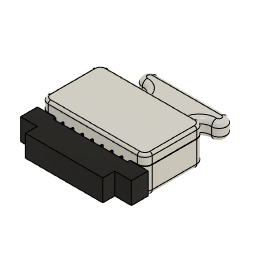
CBM8296_CP_Dongle v1 (Autodesk Fusion 360 design; units mm, degrees)
Autodesk Fusion 360 part; units mm, degrees
sketch "PCB" plane through (0, 0, 0) normal (0, 0, 1) x (1, 0, 0) in component "PCB"
  line L0 (30, 21) -> (0, 21)
  line L1 (0, 21) -> (0, 0)
  line L2 (0, 0) -> (30, 0)
  line L3 (30, 0) -> (30, 21)
  line L4 (2.87, 0) -> (2.87, -1)
  line L5 (19.05, 9.8425) -> (11.43, 9.8425)
  line L6 (7.33, -1) -> (7.33, 0)
  line L7 (25.9, 0.1) -> (25.9, -1)
  line L8 (15.98, 0.1) -> (15.98, -1)
  line L9 (-4.12, 0) -> (-5.82, 0)
  line L10 (11.43, 8.5725) -> (10.668, 8.5725)
  line L11 (14.75, 0) -> (14.75, -1)
  circle A0 centre (4, 12) radius 1.7463
  line L12 (15.25, 0) -> (14.75, 0)
  line L13 (14.02, 0.1) -> (14.02, -1)
  line L14 (23.17, 0) -> (22.67, 0)
  line L15 (8.06, 0.1) -> (8.06, -1)
  circle A1 centre (26, 12) radius 3.1789
  line L16 (3.37, 0) -> (2.87, 0)
  line L17 (19.21, -1) -> (19.21, 0)
  line L18 (10.06, 0.1) -> (10.06, -1)
  line L19 (6.1, 0.1) -> (6.1, -1)
  line L20 (0.08, -1) -> (0.08, 0)
  line L21 (-2.42, -6.8) -> (-2.42, -5.2)
  line L22 (15.25, -1) -> (15.25, 0)
  line L23 (4.1, 0.1) -> (4.1, -1)
  line L24 (19.21, 0) -> (18.71, 0)
  line L25 (26.63, 0) -> (26.63, -1)
  line L26 (18.71, 0) -> (18.71, -1)
  line L27 (29.92, -1) -> (0.08, -1)
  line L28 (-4.12, -7.9147) -> (-4.12, -8.052)
  line L29 (11.43, 9.8425) -> (11.43, 7.3025)
  line L30 (34.12, 0) -> (32.42, 0)
  line L31 (23.17, -1) -> (23.17, 0)
  line L32 (6.83, 0) -> (6.83, -1)
  line L33 (-4.12, -3.548) -> (-4.12, -3.6853)
  line L34 (23.9, 0.1) -> (23.9, -1)
  line L35 (37.37, 0) -> (35.82, 0)
  circle A2 centre (4, 12) radius 3.1789
  line L36 (12.02, 0.1) -> (12.02, -1)
  line L37 (7.33, 0) -> (6.83, 0)
  line L38 (27.13, -1) -> (27.13, 0)
  line L39 (11.29, 0) -> (10.79, 0)
  line L40 (10.79, 0) -> (10.79, -1)
  line L41 (-5.82, -6.8) -> (-7.37, -6.8)
  line L42 (11.43, 10.4775) -> (19.05, 10.4775)
  line L43 (-4.12, -4.3667) -> (-4.12, -7.2333)
  line L44 (11.29, -1) -> (11.29, 0)
  line L45 (19.94, 0.1) -> (19.94, -1)
  line L46 (27.13, 0) -> (26.63, 0)
  line L47 (3.37, -1) -> (3.37, 0)
  circle A3 centre (26, 12) radius 1.7463
  line L48 (17.98, 0.1) -> (17.98, -1)
  line L49 (37.37, 0) -> (37.37, -6.8)
  line L50 (21.94, 0.1) -> (21.94, -1)
  line L51 (22.67, 0) -> (22.67, -1)
  line L52 (35.82, -6.8) -> (32.42, -6.8)
  line L53 (0.08, 0) -> (-2.42, 0)
  line L54 (-5.82, 0) -> (-7.37, 0)
  line L55 (32.42, -4.2) -> (32.42, -2.6)
  line L56 (35.82, 0) -> (34.12, 0)
  line L57 (35.82, -4.2) -> (35.82, -2.6)
  line L58 (35.82, -6.8) -> (35.82, -5.2)
  line L59 (-4.12, 0) -> (-4.12, -2.8667)
  line L60 (30.62, -11.6) -> (-0.62, -11.6)
  line L61 (19.05, 8.5725) -> (19.812, 8.5725)
  line L62 (-0.62, -11.6) -> (-0.62, -6.8)
  line L63 (19.05, 11.7475) -> (19.812, 11.7475)
  line L64 (34.12, -3.6853) -> (34.12, -3.548)
  line L65 (34.12, -2.8667) -> (34.12, 0)
  line L66 (-2.42, -6.8) -> (-5.82, -6.8)
  line L67 (11.43, 13.0175) -> (11.43, 10.4775)
  line L68 (37.37, -6.8) -> (35.82, -6.8)
  line L69 (34.12, -11.6) -> (34.12, -8.7333)
  line L70 (11.43, 11.7475) -> (10.668, 11.7475)
  line L71 (34.12, -7.2333) -> (34.12, -4.3667)
  line L72 (-5.82, -1.6) -> (-5.82, 0)
  line L73 (-5.82, -4.2) -> (-5.82, -2.6)
  line L74 (34.12, -8.052) -> (34.12, -7.9147)
  line L75 (19.05, 10.4775) -> (19.05, 13.0175)
  line L76 (32.42, -6.8) -> (32.42, -5.2)
  line L77 (-2.42, -4.2) -> (-2.42, -2.6)
  line L78 (-7.37, 0) -> (-7.37, -6.8)
  line L79 (19.05, 7.3025) -> (19.05, 9.8425)
  line L80 (32.42, 0) -> (29.92, 0)
  line L81 (29.92, 0) -> (29.92, -1)
  line L82 (30.62, -6.8) -> (30.62, -11.6)
  line L83 (-4.12, -8.7333) -> (-4.12, -11.6)
  line L84 (35.82, -1.6) -> (35.82, 0)
  line L85 (-2.42, -1.6) -> (-2.42, 0)
  line L86 (32.42, -6.8) -> (30.62, -6.8)
  line L87 (11.43, 7.3025) -> (19.05, 7.3025)
  line L88 (-5.82, -6.8) -> (-5.82, -5.2)
  line L89 (32.42, -1.6) -> (32.42, 0)
  line L90 (-2.42, 0) -> (-4.12, 0)
  line L91 (19.05, 13.0175) -> (11.43, 13.0175)
  line L92 (-0.62, -6.8) -> (-2.42, -6.8)
  line L93 (25.9, 0.1) -> (25.9, 4)
  line L94 (25.4, 3) -> (25.4, 2)
  line L95 (4.6, 3) -> (4.6, 2)
  line L96 (6.1, 0.1) -> (6.1, 4)
  line L97 (13.52, 3) -> (13.52, 2)
  arc A4 (14.02, 4) -> (12.02, 4) centre (13.02, 4) ccw
  line L98 (17.48, 3) -> (17.48, 2)
  line L99 (10.06, 0.1) -> (10.06, 4)
  line L100 (23.9, 0.1) -> (23.9, 4)
  arc A5 (25.4, 3) -> (24.4, 3) centre (24.9, 3) ccw
  arc A6 (20.44, 2) -> (21.44, 2) centre (20.94, 2) ccw
  line L101 (21.44, 3) -> (21.44, 2)
  arc A7 (8.56, 2) -> (9.56, 2) centre (9.06, 2) ccw
  line L102 (4.1, 0.1) -> (4.1, 4)
  arc A8 (25.9, 4) -> (23.9, 4) centre (24.9, 4) ccw
  line L103 (24.4, 3) -> (24.4, 2)
  line L104 (14.02, 0.1) -> (14.02, 4)
  arc A9 (13.52, 3) -> (12.52, 3) centre (13.02, 3) ccw
  arc A10 (24.4, 2) -> (25.4, 2) centre (24.9, 2) ccw
  arc A11 (9.56, 3) -> (8.56, 3) centre (9.06, 3) ccw
  arc A12 (17.48, 3) -> (16.48, 3) centre (16.98, 3) ccw
  line L105 (16.48, 3) -> (16.48, 2)
  line L106 (9.56, 3) -> (9.56, 2)
  line L107 (17.98, 0.1) -> (17.98, 4)
  arc A13 (17.98, 4) -> (15.98, 4) centre (16.98, 4) ccw
  line L108 (12.52, 3) -> (12.52, 2)
  line L109 (19.94, 0.1) -> (19.94, 4)
  arc A14 (16.48, 2) -> (17.48, 2) centre (16.98, 2) ccw
  arc A15 (21.94, 4) -> (19.94, 4) centre (20.94, 4) ccw
  arc A16 (6.1, 4) -> (4.1, 4) centre (5.1, 4) ccw
  arc A17 (4.6, 2) -> (5.6, 2) centre (5.1, 2) ccw
  line L110 (20.44, 3) -> (20.44, 2)
  arc A18 (5.6, 3) -> (4.6, 3) centre (5.1, 3) ccw
  line L111 (8.56, 3) -> (8.56, 2)
  line L112 (5.6, 3) -> (5.6, 2)
  line L113 (12.02, 0.1) -> (12.02, 4)
  arc A19 (21.44, 3) -> (20.44, 3) centre (20.94, 3) ccw
  line L114 (8.06, 0.1) -> (8.06, 4)
  arc A20 (10.06, 4) -> (8.06, 4) centre (9.06, 4) ccw
  arc A21 (12.52, 2) -> (13.52, 2) centre (13.02, 2) ccw
  line L115 (15.98, 0.1) -> (15.98, 4)
  line L116 (21.94, 0.1) -> (21.94, 4)
extrude "Extrude1" add sketch "PCB" against normal blind 1.6 contours L0 L1 L2 L3 L7 L8 L12 L13 L14 L15 L16 L18 L19 L23 L24 L34 L36 L37 L39 L45 L46 L48 L50 L53 L80 L93 L96 A4 L99 L100 L102 A8 L104 L107 A13 L109 A15 A16 L113 L114 A20 L115 L116 | L2 L7 L34 L93 L100 A8 | L2 L19 L23 L96 L102 A16 | L2 L45 L50 L109 A15 L116 | L2 L15 L18 L99 L114 A20 | L2 L8 L48 L107 A13 L115 | L2 L13 L36 A4 L104 L113 | L5 L29 L79 L87 | A1 | A2 | L42 L67 L75 L91 | L94 A5 L103 A10 | L95 A17 A18 L112 | L97 A9 L108 A21 | L98 A12 L105 A14 | A6 L101 L110 A19 | A7 A11 L106 L111 makes body 1 in component "PCB"
extrude "Extrude9" add sketch "PCB" along normal blind 4.3 and the other way blind 4.4 contours L2 L9 L20 L27 L30 L35 L41 L49 L52 L53 L54 L56 L60 L62 L66 L68 L78 L80 L81 L82 L86 L90 L92 | L2 L25 L27 L38 L46 | L2 L4 L16 L27 L47 | L2 L14 L27 L31 L51 | L2 L6 L27 L32 L37 | L2 L17 L24 L26 L27 | L2 L27 L39 L40 L44 | L2 L11 L12 L22 L27 bodies 1 in component "PCB"
extrude "Extrude10" add sketch "PCB" along normal blind 0.5 contours L2 L7 L27 L34 | L2 L7 L34 L93 L100 A8 | L2 L19 L23 L96 L102 A16 | L2 L19 L23 L27 | L2 L27 L45 L50 | L2 L45 L50 L109 A15 L116 | L2 L15 L18 L99 L114 A20 | L2 L15 L18 L27 | L2 L8 L27 L48 | L2 L8 L48 L107 A13 L115 | L2 L13 L36 A4 L104 L113 | L2 L13 L27 L36 bodies 1 in component "PCB"
extrude "Extrude11" add sketch "PCB" against normal blind 0.5 from surface at -1.6 contours L2 L7 L27 L34 | L2 L7 L34 L93 L100 A8 | L2 L19 L23 L96 L102 A16 | L2 L19 L23 L27 | L2 L27 L45 L50 | L2 L45 L50 L109 A15 L116 | L2 L15 L18 L99 L114 A20 | L2 L15 L18 L27 | L2 L8 L27 L48 | L2 L8 L48 L107 A13 L115 | L2 L13 L36 A4 L104 L113 | L2 L13 L27 L36 bodies 1 in component "PCB"
ref_plane "WorkPlane1" through (0, 0, -4.4) normal (0, 0, 1) x (1, 0, 0) in component "bottom_shell"
sketch "bottom" plane through (0, 0, -4.4) normal (0, 0, 1) x (1, 0, 0) in component "bottom_shell"
  line L0 (15, 19.9973) -> (15, -5.0027) construction
  circle A0 centre (26, 12) radius 1.75
  circle A1 centre (4, 12) radius 1.75
  line L1 (36, 2.9752) -> (36, 20.9752)
  line L2 (-6, 2.9752) -> (-6, 20.9752)
  line L3 (33, 23.9752) -> (-3, 23.9752)
  line L4 (33, -0.0248) -> (-3, -0.0248)
  arc A2 (33, -0.0248) -> (36, 2.9752) centre (33, 2.9752) ccw
  arc A3 (36, 20.9752) -> (33, 23.9752) centre (33, 20.9752) ccw
  arc A4 (-3, 23.9752) -> (-6, 20.9752) centre (-3, 20.9752) ccw
  arc A5 (-6, 2.9752) -> (-3, -0.0248) centre (-3, 2.9752) ccw
  line L5 (33, 21.9752) -> (-3, 21.9752)
  arc A6 (-3, 21.9752) -> (-4, 20.9752) centre (-3, 20.9752) ccw
  line L6 (-4, 2.9752) -> (-4, 20.9752)
  arc A7 (-4, 2.9752) -> (-3, 1.9752) centre (-3, 2.9752) ccw
  line L7 (33, 1.9752) -> (-3, 1.9752)
  arc A8 (33, 1.9752) -> (34, 2.9752) centre (33, 2.9752) ccw
  line L8 (34, 2.9752) -> (34, 20.9752)
  arc A9 (34, 20.9752) -> (33, 21.9752) centre (33, 20.9752) ccw
  circle A10 centre (26, 12) radius 4.25
  circle A11 centre (4, 12) radius 4.25
  line L9 (30.6, 1.1752) -> (30.6, 1.9752)
  line L10 (-0.6, -0.0248) -> (-0.6, 1.9752)
  circle A12 centre (26, 12) radius 3
  circle A13 centre (4, 12) radius 3
  line L11 (33, 22.7752) -> (-3, 22.7752)
  arc A14 (-3, 22.7752) -> (-4.8, 20.9752) centre (-3, 20.9752) ccw
  line L12 (-4.8, 2.9752) -> (-4.8, 20.9752)
  arc A15 (-4.8, 2.9752) -> (-3, 1.1752) centre (-3, 2.9752) ccw
  arc A16 (33, 1.1752) -> (34.8, 2.9752) centre (33, 2.9752) ccw
  line L13 (34.8, 2.9752) -> (34.8, 20.9752)
  arc A17 (34.8, 20.9752) -> (33, 22.7752) centre (33, 20.9752) ccw
  line L14 (33, 1.1752) -> (30.6, 1.1752)
  line L15 (-0.6, 1.1752) -> (-3, 1.1752)
  line L16 (30.6, 1.1752) -> (30.6, -0.0248)
  line L17 (29, 28.9752) -> (29, 33.9752) construction
  line L18 (29, 33.9752) -> (1, 33.9752) construction
  line L19 (29, 33.9752) -> (29, 39.501) construction
  arc A18 (29, 33.9752) -> (29, 39.9752) centre (29, 36.9752) ccw
  arc A19 (29, 33.9752) -> (29, 23.9752) centre (29, 28.9752) ccw
  arc A20 (1, 23.9752) -> (1, 33.9752) centre (1, 28.9752) ccw
  line L20 (0, 21) -> (0, 0) construction
  line L21 (30, 0) -> (30, 21) construction
  line L22 (30, 21) -> (0, 21) construction
  line L23 (0, 0) -> (30, 0) construction
  circle A21 centre (26, 12) radius 1.7463 construction
  circle A22 centre (4, 12) radius 1.7463 construction
  arc A23 (1, 39.9752) -> (1, 33.9752) centre (1, 36.9752) ccw
  line L24 (1, 39.9752) -> (29, 39.9752)
  point P0 (36, 0)
  point P1 (36, 23.9752)
  point P2 (-6, -0.0248)
  point P3 (-6, 23.9752)
  dimension "d181" = 3.5
  dimension "d182" = 3.5
  dimension "d186" = 3
  dimension "d187" = 24
  dimension "d188" = 42
  dimension "d190" = 8.5
  dimension "d191" = 8.5
  dimension "d194" = 6
  dimension "d195" = 6
  dimension "d197" = 1.2
  dimension "d236" = 10
  dimension "d237" = 14
  dimension "d238" = 5
  dimension "d239" = 6
  constraint vertical L1
  constraint perpendicular L1 L3
  constraint coincident P0 L1
  constraint tangent L1 A2
  constraint tangent L4 A2
  constraint coincident P1 L1
  constraint coincident P1 L3
  constraint tangent L1 A3
  constraint tangent L3 A3
  constraint equal A2 A3
  constraint coincident P3 L2
  constraint coincident P3 L3
  constraint tangent L2 A4
  constraint tangent L3 A4
  constraint equal A2 A4
  constraint coincident P2 L2
  constraint coincident P2 L4
  constraint tangent L2 A5
  constraint tangent L4 A5
  constraint equal A2 A5
  constraint coincident L7 L9.end
  constraint perpendicular L7 L9
  constraint coincident L4 L10.start
  constraint coincident L7 L10.end
  constraint perpendicular L7 L10
  constraint parallel L3 L11
  constraint concentric A4 A14
  constraint parallel L2 L12
  constraint concentric A5 A15
  constraint parallel L4 L14
  constraint concentric A2 A16
  constraint parallel L1 L13
  constraint concentric A3 A17
  constraint tangent L11 A17
  constraint tangent A14 L12
  constraint tangent L11 A14
  constraint tangent L13 A17
  constraint tangent L12 A15
  constraint tangent A15 L14
  constraint tangent A16 L14
  constraint tangent A16 L13
  constraint collinear L14 L15
  constraint coincident L10 L15.start
  constraint coincident L4 L16.end
  constraint perpendicular L4 L16
  constraint coincident L17.start A19.centre
  constraint vertical L17
  constraint tangent L18 A20
  constraint tangent L18 A18
  constraint perpendicular L18 L19
  constraint coincident A18.centre L19
  constraint coincident L19 A18.end
  constraint coincident L3 A19.end
  constraint coincident L3 A20.start
  constraint symmetric L0 L20 L21
  constraint concentric A1 A22
  constraint concentric A1 A13
  constraint concentric A1 A11
  constraint concentric A10 A21
  constraint concentric A12 A21
  constraint concentric A0 A21
  constraint symmetric L0 L1 L2
  constraint symmetric L0 A19 A20
  constraint symmetric L0 L17.end L18.end
  constraint symmetric L0 A18.end A23.start
  constraint symmetric L0 A18 A23
  measures "d181" diameter of A0
  measures "d182" diameter of A1
  measures "d186" radius of A2
  measures "d187" distance of L3 L4
  measures "d188" distance of L1 L2
  measures "d190" diameter of A10
  measures "d191" diameter of A11
  measures "d194" diameter of A12
  measures "d195" diameter of A13
  measures "d197" distance of L3 L11
  measures "d236" diameter of A19
  measures "d237" distance of L0 L17.start
  measures "d238" distance of L3 L17.start
  measures "d239" diameter of A18
extrude "Extrude1'" add sketch "bottom" against normal blind 2 separate body contours L1 L2 L3 L4 A2 A3 A4 A5 L10 L11 A14 L12 A15 A16 L13 A17 L14 L15 L16 | L4 L7 L9 L10 L16 | L3 A18 A19 A20 A23 L24 | L5 A6 L6 A7 L7 A8 L8 A9 L9 L10 L11 A14 L12 A15 A16 L13 A17 L14 L15 | L5 A6 L6 A7 L7 A8 L8 A9 | A10 | A11 makes body 2 in component "bottom_shell"
extrude "Extrude2" add sketch "bottom" along normal blind 2.8 contours A10 | A11 | A12 | A13 bodies 2 in component "bottom_shell"
extrude "Extrude3" add sketch "bottom" along normal blind 1.8 contours L4 L7 L9 L10 L16 bodies 2 in component "bottom_shell"
extrude "Extrude4" add sketch "bottom" along normal blind 9.7 contours L5 A6 L6 A7 L7 A8 L8 A9 L9 L10 L11 A14 L12 A15 A16 L13 A17 L14 L15 bodies 2 in component "bottom_shell"
extrude "Extrude5" add sketch "bottom" along normal blind 8.7 contours L1 L2 L3 L4 A2 A3 A4 A5 L10 L11 A14 L12 A15 A16 L13 A17 L14 L15 L16 bodies 2 in component "bottom_shell"
extrude "Extrude6" add sketch "bottom" along normal blind 5 contours L3 A18 A19 A20 A23 L24 bodies 2 in component "bottom_shell"
fillet "Fillet1" radius 1 8 edges at (15, 1.9752, -4.4) (33.7071, 2.2681, -4.4) (34, 11.9752, -4.4) (33.7071, 21.6823, -4.4) (15, 21.9752, -4.4) (-3.7071, 21.6823, -4.4) (-4, 11.9752, -4.4) (-3.7071, 2.2681, -4.4) on bodies 2 in component "bottom_shell"
fillet "Fillet2" radius 1 2 edges at (0.0376, 13.5369, -4.4) (22.0376, 13.5369, -4.4) on bodies 2 in component "bottom_shell"
chamfer "Chamfer1" distance 1 angle 45 2 edges at (0.0376, 10.4631, -1.6) (22.0376, 10.4631, -1.6) on bodies 2 in component "bottom_shell"
fillet "Fillet5" radius 2 19 edges at (15, -0.0248, -6.4) (-5.1213, 0.8538, -6.4) (-6, 11.9752, -6.4) (-5.1213, 23.0965, -6.4) (-1, 23.9752, -6.4) (6, 28.9752, -6.4) (-2, 36.9752, -6.4) (15, 39.9752, -6.4) (32, 36.9752, -6.4) (24, 28.9752, -6.4) (31, 23.9752, -6.4) (35.1213, 23.0965, -6.4) (36, 11.9752, -6.4) (35.1213, 0.8538, -6.4) (24, 28.9752, 0.6) (32, 36.9752, 0.6) (15, 39.9752, 0.6) (-2, 36.9752, 0.6) (6, 28.9752, 0.6) on bodies 2 in component "bottom_shell"
fillet "Fillet6" radius 0.5 2 edges at (-0.6, 0.9752, -2.6) (30.6, 0.9752, -2.6) on bodies 2 in component "bottom_shell"
ref_plane "WorkPlane1" through (0, 0, 6.5) normal (0, 0, 1) x (1, 0, 0) in component "top_shell"
sketch "top" plane through (0, 0, 6.5) normal (0, 0, 1) x (1, 0, 0) in component "top_shell"
  line L0 (33, 23.9752) -> (-3, 23.9752)
  arc A0 (-3, 23.9752) -> (-6, 20.9752) centre (-3, 20.9752) ccw
  line L1 (-6, 2.9752) -> (-6, 20.9752)
  arc A1 (-6, 2.9752) -> (-3, -0.0248) centre (-3, 2.9752) ccw
  line L2 (33, -0.0248) -> (-3, -0.0248)
  line L3 (33, 1.9752) -> (-3, 1.9752)
  arc A2 (-4, 2.9752) -> (-3, 1.9752) centre (-3, 2.9752) ccw
  line L4 (-4, 2.9752) -> (-4, 20.9752)
  arc A3 (-3, 21.9752) -> (-4, 20.9752) centre (-3, 20.9752) ccw
  line L5 (33, 21.9752) -> (-3, 21.9752)
  line L6 (34, 2.9752) -> (34, 20.9752)
  arc A4 (34, 20.9752) -> (33, 21.9752) centre (33, 20.9752) ccw
  arc A5 (33, 1.9752) -> (34, 2.9752) centre (33, 2.9752) ccw
  arc A6 (33, -0.0248) -> (36, 2.9752) centre (33, 2.9752) ccw
  line L7 (36, 2.9752) -> (36, 20.9752)
  arc A7 (36, 20.9752) -> (33, 23.9752) centre (33, 20.9752) ccw
  line L8 (-0.6, -0.0248) -> (-0.6, 1.9752)
  line L9 (30.6, 1.1752) -> (30.6, -0.0248)
  line L10 (30.6, 1.1752) -> (30.6, 1.9752)
  circle A8 centre (4, 12) radius 1.75 construction
  circle A9 centre (26, 12) radius 1.75 construction
  circle A10 centre (4, 12) radius 1.25
  circle A11 centre (26, 12) radius 1.25
  circle A12 centre (4, 12) radius 3.5
  circle A13 centre (26, 12) radius 3.5
  line L11 (35.2, 2.9752) -> (35.2, 20.9752)
  arc A14 (35.2, 20.9752) -> (33, 23.1752) centre (33, 20.9752) ccw
  line L12 (33, 23.1752) -> (-3, 23.1752)
  arc A15 (-3, 23.1752) -> (-5.2, 20.9752) centre (-3, 20.9752) ccw
  line L13 (-5.2, 2.9752) -> (-5.2, 20.9752)
  arc A16 (-5.2, 2.9752) -> (-3, 0.7752) centre (-3, 2.9752) ccw
  arc A17 (33, 0.7752) -> (35.2, 2.9752) centre (33, 2.9752) ccw
  line L14 (33, 0.7752) -> (30.6, 0.7752)
  line L15 (-0.6, 0.7752) -> (-3, 0.7752)
  dimension "d213" = 2.5
  dimension "d214" = 2.5
  dimension "d220" = 7
  dimension "d221" = 7
  dimension "d223" = 0.8
  constraint concentric A8 A10
  constraint concentric A9 A11
  constraint concentric A10 A12
  constraint concentric A11 A13
  constraint parallel L7 L11
  constraint concentric A7 A14
  constraint parallel L0 L12
  constraint concentric A0 A15
  constraint parallel L1 L13
  constraint concentric A1 A16
  constraint parallel L2 L14
  constraint concentric A6 A17
  constraint tangent L13 A16
  constraint tangent L11 A17
  constraint tangent A16 L14
  constraint tangent L11 A14
  constraint tangent A14 L12
  constraint tangent L12 A15
  constraint tangent A15 L13
  constraint tangent A17 L14
  constraint coincident L9 L14.end
  constraint coincident L8 L15.start
  constraint collinear L14 L15
  measures "d213" diameter of A10
  measures "d214" diameter of A11
  measures "d220" diameter of A12
  measures "d221" diameter of A13
  measures "d223" distance of L0 L12
extrude "Extrude1''" add sketch "top" along normal blind 2 separate body contours L0 A0 L1 A1 L2 A6 L7 A7 L8 L9 L11 A14 L12 A15 L13 A16 A17 L14 L15 | L2 L3 L8 L9 L10 | L3 A2 L4 A3 L5 L6 A4 A5 L8 L9 L10 L11 A14 L12 A15 L13 A16 A17 L14 L15 | L3 A2 L4 A3 L5 L6 A4 A5 | A10 | A11 | A12 | A13 makes body 3 in component "top_shell"
extrude "Extrude2'" add sketch "top" against normal blind 6.3 contours A12 | A13 bodies 3 in component "top_shell"
extrude "Extrude3'" add sketch "top" against normal blind 1 contours L3 A2 L4 A3 L5 L6 A4 A5 L8 L9 L10 L11 A14 L12 A15 L13 A16 A17 L14 L15 bodies 3 in component "top_shell"
extrude "Extrude4'" add sketch "top" against normal blind 3.5 contours L2 L3 L8 L9 L10 bodies 3 in component "top_shell"
extrude "Extrude5'" add sketch "top" against normal blind 2 contours L0 A0 L1 A1 L2 A6 L7 A7 L8 L9 L11 A14 L12 A15 L13 A16 A17 L14 L15 bodies 3 in component "top_shell"
fillet "Fillet1'" radius 1 10 edges at (15, 21.9752, 6.5) (33.7071, 21.6823, 6.5) (34, 11.9752, 6.5) (33.7071, 2.2681, 6.5) (15, 1.9752, 6.5) (-3.7071, 2.2681, 6.5) (-4, 11.9752, 6.5) (-3.7071, 21.6823, 6.5) (0.7369, 10.7343, 6.5) (22.7369, 10.7343, 6.5) on bodies 3 in component "top_shell"
fillet "Fillet2'" radius 1 8 edges at (-6, 11.9752, 8.5) (-5.1213, 0.8538, 8.5) (15, -0.0248, 8.5) (35.1213, 0.8538, 8.5) (36, 11.9752, 8.5) (35.1213, 23.0965, 8.5) (15, 23.9752, 8.5) (-5.1213, 23.0965, 8.5) on bodies 3 in component "top_shell"
component "PCB" placed x (1, 0, 0) y (0, 1, 0) z (0, 0, 1) at (0, 0, 0)
component "bottom_shell" placed x (1, 0, 0) y (0, 1, 0) z (0, 0, 1) at (0, 0, 0)
component "top_shell" placed x (1, 0, 0) y (0, 1, 0) z (0, 0, 1) at (0, 0, 0)
equation "pcb_thickness = 1.6 mm"
equation "below = 2.8 mm + pcb_thickness"
equation "wall = 2 mm"
equation "width = pcb_width + 2 mm + 2 * r_corner + 2 * wall"
equation "length = pcb_length + 1 mm + wall"
equation "above = 8.5 mm - wall"
equation "pcb_width = 30 mm"
equation "pcb_length = 21 mm"
equation "r_corner = 3 mm"
equation "drill = 3.5 mm"
equation "d_screw = 7 mm"
equation "tol_x = 0.3 mm"
equation "tol_connector = 0.6 mm"
equation "d_post = 8.5 mm"
equation "d_post2 = 8 mm"
equation "bottom_height = 4.3 mm + below"
equation "overlap = 1 mm"
equation "top_height = above + below - bottom_height - tol_y"
equation "d35 = tol_connector"
equation "d37 = d35"
equation "tol_y = 0.2 mm"
equation "d154 = -pcb_thickness"
equation "d176 = -pcb_thickness"
equation "d180 = -below"
equation "d181 = drill"
equation "d182 = drill"
equation "d186 = r_corner"
equation "d187 = length"
equation "d188 = width"
equation "d189 = -wall"
equation "d190 = d_post"
equation "d191 = d_post"
equation "d195 = d194"
equation "d197 = 0.6 * wall"
equation "d198 = -wall"
equation "d200 = below - pcb_thickness"
equation "d202 = below - pcb_thickness - 1 mm"
equation "d204 = bottom_height + overlap"
equation "d206 = bottom_height"
equation "d212 = above"
equation "d220 = d_screw"
equation "d221 = d_screw"
equation "d223 = 0.4 * wall"
equation "d224 = wall"
equation "d226 = -above + tol_y"
equation "d228 = -top_height + overlap"
equation "d230 = -top_height - 1.5 mm"
equation "d232 = -top_height"
equation "d238 = d236 / 2"
named bodies: "PCB", "bottom", "top"
